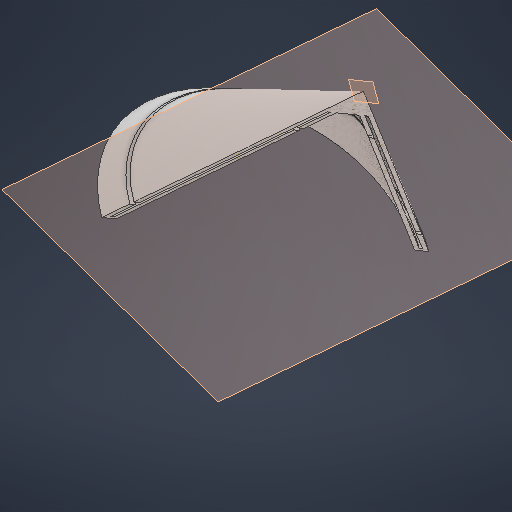
# Autodesk Inventor part: Tree Model-Om Mihani
Saved by Autodesk Inventor 2026.2 (Build 302298000, 298)
## iProperties
Created: 2026-08-23
Part Number: Tree Model-Om Mihani
Material: Generic
Document SubType Name: Modeling
Designer: Atharva Bapat
Density: 1 g/cm^3
Appearance: Default
Author: Atharva Bapat
Autodesk Inventor part; units mm, degrees
ref_plane "YZ Plane" through (0, 0, 0) normal (1, 0, 0) x (0, 1, 0)
ref_plane "XZ Plane" through (0, 0, 0) normal (0, 1, 0) x (-1, 0, 0)
ref_plane "XY Plane" through (0, 0, 0) normal (0, 0, 1) x (1, 0, 0)
sketch "Sketch1" plane through (0, 0, 0) normal (1, 0, 0) x (0, 1, 0)
  line L0 (0, 0) -> (150, 0)
  line L1 (150, 0) -> (-150, 0)
  line L2 (0, 0) -> (-100, 0)
  line L3 (-100, 0) -> (-100, 150)
  line L4 (-100, 0) -> (-95, 0)
  line L5 (63.1336, 18.679) -> (63.1336, 0)
  line L6 (-95, 141.128) -> (-95, 138.128)
  line L7 (63.1336, 15.679) -> (63.1336, 10.679)
  line L8 (63.1336, 10.679) -> (39.4136, 29.0464)
  line L9 (-100, 150) -> (-76.9079, 132.1189)
  line L10 (-73.9079, 129.7959) -> (93.7137, 0)
  line L11 (-95, 141.128) -> (-76.9079, 127.1186)
  line L12 (-73.9079, 124.7956) -> (63.1336, 18.679)
  line L13 (-73.9079, 129.7959) -> (-73.9079, 124.7956)
  line L14 (-76.9079, 129.7959) -> (-76.9079, 127.1186)
  line L15 (-76.9079, 127.1186) -> (-76.9079, 132.1189)
  line L16 (-95, 138.128) -> (36.4136, 36.3694)
  line L17 (39.4136, 34.0464) -> (63.1336, 15.679)
  line L18 (36.4136, 36.3694) -> (36.4136, 31.3694)
  line L19 (39.4136, 29.0464) -> (39.4136, 34.0464)
  line L20 (39.4136, 29.0464) -> (39.4136, 34.0464)
  line L21 (63.1336, 10.679) -> (39.4136, 29.0464)
  line L22 (36.4136, 31.3694) -> (-95, 133.128)
  line L23 (-95, 141.128) -> (-95, 146.1283)
  line L24 (-100, 150) -> (-95, 146.1283)
  line L25 (-95, 146.1283) -> (-96.8631, 147.571)
  line L26 (-95, 146.1283) -> (-97.372, 147.965)
  line L27 (-97.372, 147.965) -> (-97.5, 135.0638)
  line L28 (-97.5, 135.0638) -> (-95, 133.128)
  line L29 (-95, 141.128) -> (-95, 138.128)
  line L30 (-95, 141.128) -> (-95, 138.128)
  line L31 (-95, 0) -> (-95, 133.128)
  line L32 (-95, 138.128) -> (-95, 141.128)
  dimension "d0" = 150
  dimension "d1" = 300
  dimension "d2" = 100
  dimension "d3" = 150
  dimension "d4" = 245
  dimension "d5" = 5
  dimension "d6" = 141.128
  dimension "d7" = 200
  dimension "d8" = 3
  dimension "d9" = 5
  dimension "d12" = 30
  dimension "d15" = 3
  constraints: 66 end point, 10 parallel, 10 point on line, 4 collinear, 4 perpendicular, 1 horizontal, 1 vertical
  measures "d0" distance of L0.start L0.end
  measures "d1" distance of L0.end L1.end
  measures "d2" distance of L0.start L2.end
  measures "d3" distance of L2.end L3.end
  measures "d4" distance of L3.end L10.end
  measures "d5" distance of L2.end L4.end
  measures "d6" distance of L6.start L4.end
  measures "d7" distance of L6.start L5.start
  measures "d8" distance of L6.end L6.start
  measures "d9" distance of L7.start L7.end
  measures "d12" distance of L7.end L8.end
  measures "d15" distance of L23.end L26.end
ref_plane "Work Plane1" through (0, 93.7137, 0) normal (0, 1, 0) x (-1, 0, 0)
ref_plane "Work Plane2" through (0, 93.7137, 0) normal (1, 0, 0) x (0, -0.7907, 0.6122)
revolve "Revolution1" add sketch "Sketch1" angle 360 about axis through (0, 0, 0) along (0, -1, 0) contours L5 L12 L13 L10 L0 | L8 L19 L17 L5 | L28 L27 L9 L23 L6 L16 L18 L22 | L9 L15 L14 L11 L23
body "Solid1"
